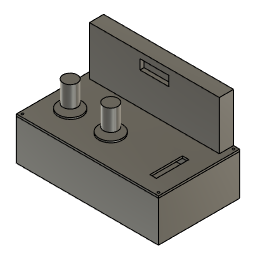
enclosure v8 (Autodesk Fusion 360 design; units mm, degrees)
Autodesk Fusion 360 part; units mm, degrees
note: some values were not read from the file. Set by a fixed rule: which face or edge a step refers to.
sketch "Sketch1" plane through (0, 0, 0) normal (0, 0, 1) x (1, 0, 0) in component "base"
  line L0 (175, 100) -> (-175, 100)
  line L1 (-175, 100) -> (-175, -100)
  line L2 (-175, -100) -> (175, -100)
  line L3 (175, -100) -> (175, 100)
  line L4 (175, 100) -> (-175, -100) construction
  line L5 (-175, 100) -> (175, -100) construction
  dimension "d1" = 350
  dimension "d2" = 200
  constraint horizontal L0
  constraint perpendicular L0 L1
  constraint parallel L0 L2
  constraint parallel L1 L3
  constraint coincident L4 origin
  constraint coincident L5 origin
  measures "d1" distance of L1.end L2.end
  measures "d2" distance of L0.end L1.end
extrude "Extrude1" add sketch "Sketch1" along normal blind 100 makes body 1 in component "base"
sketch "Sketch2" plane through (0, 0, 100) normal (0, 0, 1) x (-1, 0, 0) in component "base"
  line L0 (-175, 100) -> (-175, -100)
  line L1 (-175, -100) -> (175, -100)
  line L2 (175, -100) -> (175, 100)
  line L3 (175, 100) -> (-175, 100)
  line L4 (-160, -85) -> (160, -85)
  line L5 (160, -85) -> (160, 85)
  line L6 (160, 85) -> (-160, 85)
  line L7 (-160, 85) -> (-160, -85)
  line L8 (-160, -85) -> (160, 85) construction
  line L9 (160, -85) -> (-160, 85) construction
  dimension "d5" = 15
  dimension "d6" = 15
  constraint horizontal L4
  constraint perpendicular L4 L5
  constraint parallel L4 L6
  constraint parallel L5 L7
  constraint coincident L8 origin
  constraint coincident L9 origin
  measures "d5" distance of L0 L7
  measures "d6" distance of L3 L6
extrude "Extrude2" cut sketch "Sketch2" against normal up to surface (85 mm away) contours L4 L5 L6 L7 bodies 1 in component "base"
sketch "Sketch3" plane through (0, 0, 100) normal (0, 0, 1) x (-1, 0, 0) in component "base"
  line L0 (-160, 85) -> (160, 85)
  line L1 (160, 85) -> (160, -85)
  line L2 (160, -85) -> (-160, -85)
  line L3 (-160, -85) -> (-160, 85)
  line L4 (-175, 100) -> (-175, -100)
  line L5 (-175, -100) -> (175, -100)
  line L6 (175, -100) -> (175, 100)
  line L7 (175, 100) -> (-175, 100)
  circle A0 centre (-167.5, -92.5) radius 2.5
  dimension "d9" = 7.5
  dimension "d10" = 7.5
  dimension "d11" = 5
  measures "d9" distance of L5 A0.centre
  measures "d10" distance of L4 A0.centre
  measures "d11" diameter of A0
extrude "Extrude3" cut sketch "Sketch3" against normal blind 10 contours A0 bodies 1 in component "base"
mirror "Mirror1" about plane through (0, 0, 0) normal (1, 0, 0) of "Extrude3" in component "base"
mirror "Mirror2" about plane through (0, 0, 0) normal (0, 1, 0) of "Extrude3", "Mirror1" in component "base"
sketch "Sketch1 (2)" plane through (0, 0, 100) normal (0, 0, 1) x (-1, 0, 0) in component "lid"
  circle A0 centre (167.5, 92.5) radius 2.5
  circle A1 centre (-167.5, 92.5) radius 2.5
  circle A2 centre (167.5, -92.5) radius 2.5
  circle A3 centre (-167.5, -92.5) radius 2.5
  line L0 (-160, 85) -> (160, 85)
  line L1 (160, 85) -> (160, -85)
  line L2 (160, -85) -> (-160, -85)
  line L3 (-160, -85) -> (-160, 85)
  line L4 (-175, 100) -> (-175, -100)
  line L5 (-175, -100) -> (175, -100)
  line L6 (175, -100) -> (175, 100)
  line L7 (175, 100) -> (-175, 100)
  line L8 (-175, -100) -> (175, -100)
  line L9 (175, -100) -> (175, 100)
  line L10 (175, 100) -> (-175, 100)
  line L11 (-175, 100) -> (-175, -100)
  line L12 (-175, -100) -> (175, 100) construction
  line L13 (175, -100) -> (-175, 100) construction
  constraint horizontal L8
  constraint perpendicular L8 L9
  constraint parallel L8 L10
  constraint parallel L9 L11
  constraint coincident L12 origin
  constraint coincident L13 origin
  constraint coincident L4.end L5.start
  measures "d109" distance of L4.start
extrude "Extrude1'" add sketch "Sketch1 (2)" along normal blind 5 separate body contours L0 L1 L2 L3 | L4 L5 L6 L7 L8 L9 L10 L11 makes body 2 in component "lid"
sketch "Sketch2 (2)" plane through (0, 0, 105) normal (0, 0, 1) x (-1, 0, 0) in component "lid"
  circle A0 centre (-167.5, -92.5) radius 2.5
  circle A1 centre (167.5, -92.5) radius 2.5
  circle A2 centre (167.5, 92.5) radius 2.5
  circle A3 centre (-167.5, 92.5) radius 2.5
  line L0 (-175, 100) -> (-175, -100)
  line L1 (-175, -100) -> (175, -100)
  line L2 (175, -100) -> (175, 100)
  line L3 (175, 100) -> (-175, 100)
  circle A4 centre (117.5, 25) radius 17.5
  dimension "d20" = 75
  dimension "d21" = 57.5
  dimension "d22" = 35
  measures "d20" distance of L3 A4.centre
  measures "d21" distance of L2 A4.centre
  measures "d22" diameter of A4
extrude "Extrude2'" cut sketch "Sketch2 (2)" against normal blind 5 contours A4 bodies 2 in component "lid"
sketch "Sketch3 (2)" plane through (0, 0, 105) normal (0, 0, 1) x (-1, 0, 0) in component "lid"
  circle A0 centre (117.5, 25) radius 17.5
  circle A1 centre (-167.5, -92.5) radius 2.5
  circle A2 centre (167.5, -92.5) radius 2.5
  circle A3 centre (167.5, 92.5) radius 2.5
  circle A4 centre (-167.5, 92.5) radius 2.5
  line L0 (-175, 100) -> (-175, -100)
  line L1 (-175, -100) -> (175, -100)
  line L2 (175, -100) -> (175, 100)
  line L3 (175, 100) -> (-175, 100)
  circle A5 centre (17.5, 25) radius 17.5
  line L4 (175, 100) -> (-175, 100)
  dimension "d25" = 35
  dimension "d26" = 100
  dimension "d33" = 75
  measures "d25" diameter of A5
  measures "d26" distance of A0.centre A5.centre
  measures "d33" distance of A5.centre L4
extrude "Extrude3'" cut sketch "Sketch3 (2)" against normal blind 5 contours A5 bodies 2 in component "lid"
sketch "Sketch4" plane through (0, 0, 105) normal (0, 0, 1) x (-1, 0, 0) in component "lid"
  circle A0 centre (17.5, 25) radius 17.5
  circle A1 centre (117.5, 25) radius 17.5
  circle A2 centre (-167.5, -92.5) radius 2.5
  circle A3 centre (167.5, -92.5) radius 2.5
  circle A4 centre (167.5, 92.5) radius 2.5
  circle A5 centre (-167.5, 92.5) radius 2.5
  line L0 (-175, 100) -> (-175, -100)
  line L1 (-175, -100) -> (175, -100)
  line L2 (175, -100) -> (175, 100)
  line L3 (175, 100) -> (-175, 100)
  line L4 (-135, 65) -> (-119, 65)
  line L5 (-119, 65) -> (-119, -15)
  line L6 (-119, -15) -> (-135, -15)
  line L7 (-135, -15) -> (-135, 65)
  line L8 (-135, 65) -> (-119, -15) construction
  line L9 (-119, 65) -> (-135, -15) construction
  point P0 (-127, 25)
  dimension "d29" = 40
  dimension "d30" = 80
  dimension "d31" = 16
  dimension "d32" = 35
  constraint horizontal L4
  constraint perpendicular L4 L5
  constraint parallel L4 L6
  constraint parallel L5 L7
  constraint coincident L8 P0
  constraint coincident L9 P0
  measures "d29" distance of L0 L7
  measures "d30" distance of L4.start L6.end
  measures "d31" distance of L5.end L6.end
  measures "d32" distance of L3 L4
extrude "Extrude4" cut sketch "Sketch4" against normal up to surface (5 mm away) contours L4 L5 L6 L7 bodies 2 in component "lid"
sketch "Sketch1 (3)" plane through (0, 0, 105) normal (0, 0, 1) x (-1, 0, 0) in component "display"
  line L0 (-119, -15) -> (-135, -15)
  line L1 (-135, -15) -> (-135, 65)
  line L2 (-135, 65) -> (-119, 65)
  line L3 (-119, 65) -> (-119, -15)
  circle A0 centre (17.5, 25) radius 17.5
  circle A1 centre (117.5, 25) radius 17.5
  circle A2 centre (167.5, 92.5) radius 2.5
  circle A3 centre (-167.5, 92.5) radius 2.5
  circle A4 centre (167.5, -92.5) radius 2.5
  circle A5 centre (-167.5, -92.5) radius 2.5
  line L4 (-175, 100) -> (-175, -100)
  line L5 (-175, -100) -> (175, -100)
  line L6 (175, -100) -> (175, 100)
  line L7 (175, 100) -> (-175, 100)
  line L8 (160, -85) -> (-160, -85)
  line L9 (0, 130) -> (0, -130) construction
  line L10 (-160, -100) -> (160, -100)
  line L11 (160, -100) -> (160, -65)
  line L12 (160, -65) -> (-160, -65)
  line L13 (-160, -65) -> (-160, -100)
  line L14 (-160, -100) -> (160, -65) construction
  line L15 (160, -100) -> (-160, -65) construction
  point P0 (0, -82.5)
  dimension "d36" = 35
  dimension "d37" = 320
  constraint perpendicular L8 L9
  constraint horizontal L10
  constraint perpendicular L10 L11
  constraint parallel L10 L12
  constraint parallel L11 L13
  constraint coincident L14 P0
  constraint coincident L15 P0
  constraint coincident L5 L10.start
  constraint coincident L9 P0
  measures "d36" distance of L10.start L12.end
  measures "d37" distance of L11.end L12.end
extrude "Extrude1''" add sketch "Sketch1 (3)" along normal blind 120 separate body contours L5 L8 L10 L11 L13 | L8 L11 L12 L13 makes body 3 in component "display"
sketch "Sketch1 (4)" plane through (0, 0, 105) normal (0, 0, 1) x (-1, 0, 0) in component "joystick"
  line L0 (-119, -15) -> (-135, -15)
  line L1 (-135, -15) -> (-135, 65)
  line L2 (-135, 65) -> (-119, 65)
  line L3 (-119, 65) -> (-119, -15)
  circle A0 centre (17.5, 25) radius 17.5
  circle A1 centre (117.5, 25) radius 17.5
  circle A2 centre (167.5, 92.5) radius 2.5
  circle A3 centre (-167.5, 92.5) radius 2.5
  circle A4 centre (167.5, -92.5) radius 2.5
  circle A5 centre (-167.5, -92.5) radius 2.5
  line L4 (-175, 100) -> (-175, -100)
  line L5 (-175, -100) -> (175, -100)
  line L6 (175, -100) -> (175, 100)
  line L7 (175, 100) -> (-175, 100)
  circle A6 centre (117.5, 25) radius 29
  dimension "d44" = 58
  constraint concentric A1 A6
  measures "d44" diameter of A6
extrude "Extrude1'''" add sketch "Sketch1 (4)" along normal blind 4 separate body contours A1 | A6 makes body 4 in component "joystick"
sketch "Sketch2 (3)" plane through (0, 0, 109) normal (0, 0, 1) x (-1, 0, 0) in component "joystick"
  circle A0 centre (117.5, 25) radius 29
  circle A1 centre (117.5, 25) radius 3
  dimension "d47" = 6
  constraint concentric A0 A1
  measures "d47" diameter of A1
extrude "Extrude2''" add sketch "Sketch2 (3)" along normal blind 10 contours A1 bodies 4 in component "joystick"
sketch "Sketch3 (3)" plane through (0, 0, 119) normal (0, 0, 1) x (-1, 0, 0) in component "joystick"
  circle A0 centre (117.5, 25) radius 3
  circle A1 centre (117.5, 25) radius 17.5
  dimension "d50" = 35
  constraint concentric A0 A1
  measures "d50" diameter of A1
extrude "Extrude3''" add sketch "Sketch3 (3)" along normal blind 52 contours A0 | A1 bodies 4 in component "joystick"
sketch "Sketch2 (4)" plane through (0, 100, 0) normal (0, 1, 0) x (-1, 0, 0) in component "display"
  line L0 (-160, 105) -> (160, 105)
  line L1 (160, 105) -> (160, 225)
  line L2 (160, 225) -> (-160, 225)
  line L3 (-160, 225) -> (-160, 105)
  line L4 (0, 90) -> (0, 250) construction
  line L5 (145, 220) -> (-145, 220)
  line L6 (-145, 220) -> (-145, 120)
  line L7 (-145, 120) -> (145, 120)
  line L8 (145, 120) -> (145, 220)
  line L9 (145, 220) -> (-145, 120) construction
  line L10 (-145, 220) -> (145, 120) construction
  point P0 (0, 170)
  dimension "d61" = 15
  dimension "d62" = 15
  dimension "d63" = 15
  dimension "d128" = 100
  constraint perpendicular L2 L4
  constraint horizontal L5
  constraint perpendicular L5 L6
  constraint parallel L5 L7
  constraint parallel L6 L8
  constraint coincident L9 P0
  constraint coincident L10 P0
  constraint midpoint L4 P0
  measures "d61" distance of L1 L8
  measures "d62" distance of L3 L6
  measures "d63" distance of L0 L7
  measures "d128" distance of L5.end L6.end
extrude "Extrude2'''" cut sketch "Sketch2 (4)" against normal up to surface (25 mm away) contours L5 L6 L7 L8 bodies 3 in component "display"
sketch "Sketch3 (4)" plane through (0, 75, 0) normal (0, 1, 0) x (-1, 0, 0) in component "display"
  line L0 (145, 220) -> (-145, 220)
  line L1 (-145, 220) -> (-145, 120)
  line L2 (-145, 120) -> (145, 120)
  line L3 (145, 120) -> (145, 220)
  line L4 (0, 80) -> (0, 240) construction
  line L5 (35.5, 210) -> (-35.5, 210)
  line L6 (-35.5, 210) -> (-35.5, 186)
  line L7 (-35.5, 186) -> (35.5, 186)
  line L8 (35.5, 186) -> (35.5, 210)
  line L9 (35.5, 210) -> (-35.5, 186) construction
  line L10 (-35.5, 210) -> (35.5, 186) construction
  point P0 (0, 198)
  dimension "d67" = 10
  dimension "d68" = 24
  dimension "d69" = 71
  constraint vertical L4
  constraint horizontal L5
  constraint perpendicular L5 L6
  constraint parallel L5 L7
  constraint parallel L6 L8
  constraint coincident L9 P0
  constraint coincident L10 P0
  constraint coincident L4 P0
  measures "d67" distance of L0 L5
  measures "d68" distance of L5.end L6.end
  measures "d69" distance of L5.start L5.end
extrude "Extrude3'''" cut sketch "Sketch3 (4)" against normal up to surface (10 mm away) contours L5 L6 L7 L8 bodies 3 in component "display"
sketch "Sketch5" plane through (0, 100, 0) normal (0, 1, 0) x (-1, 0, 0)
  line L0 (145, 120) -> (-145, 120)
  line L1 (-145, 120) -> (-145, 220)
  line L2 (-145, 220) -> (145, 220)
  line L3 (145, 220) -> (145, 120)
  line L4 (-160, 105) -> (160, 105)
  line L5 (160, 105) -> (160, 225)
  line L6 (160, 225) -> (-160, 225)
  line L7 (-160, 225) -> (-160, 105)
  line L8 (-35.5, 186) -> (-35.5, 210)
  line L9 (-47.4876, 205) -> (45, 205) construction
  line L10 (-35.5, 210) -> (14.5, 210)
  line L11 (14.5, 210) -> (14.5, 227)
  line L12 (14.5, 227) -> (-35.5, 227)
  line L13 (-35.5, 227) -> (-35.5, 210)
  dimension "d76" = 50
  dimension "d77" = 17
  constraint perpendicular L8 L9
  constraint horizontal L10
  constraint vertical L11
  constraint horizontal L12
  constraint vertical L13
  constraint coincident L8.end L10.start
  measures "d76" distance of L11.end L12.end
  measures "d77" distance of L10.end L11.end
sketch "Sketch6" plane through (0, 75, 0) normal (0, 1, 0) x (-1, 0, 0)
  line L0 (-35.5, 186) -> (-35.5, 210)
  line L1 (-145, 220) -> (-145, 120)
  line L2 (-145, 120) -> (145, 120)
  line L3 (145, 120) -> (145, 220)
  line L4 (145, 220) -> (-145, 220)
  line L5 (-35.5, 210) -> (35.5, 210)
  line L6 (35.5, 210) -> (35.5, 186)
  line L7 (35.5, 186) -> (-35.5, 186)
  circle A0 centre (37.5, 213) radius 1.5
  dimension "d80" = 2
  dimension "d81" = 3
  dimension "d82" = 3
  measures "d80" distance of L6 A0.centre
  measures "d81" distance of L5 A0.centre
  measures "d82" diameter of A0
extrude "Extrude5" cut sketch "Sketch6" against normal up to surface (5 mm away) contours A0 bodies 3 in component "display"
ref_plane "WorkPlane1" through (0, 70, 198) normal (0, 0, 1) x (-1, 0, 0)
mirror "Mirror1'" about plane through (0, 70, 198) normal (0, 0, 1) of "Extrude5" in component "display"
mirror "Mirror2'" about plane through (0, 0, 0) normal (1, 0, 0) of "Extrude5", "Mirror1'" in component "display"
sketch "Sketch4 (2)" plane through (0, 0, 100) normal (0, 0, 1) x (-1, 0, 0) in component "base"
  circle A0 centre (167.5, 92.5) radius 2.5
  circle A1 centre (-167.5, 92.5) radius 2.5
  circle A2 centre (167.5, -92.5) radius 2.5
  circle A3 centre (-167.5, -92.5) radius 2.5
  line L0 (-160, 85) -> (160, 85)
  line L1 (160, 85) -> (160, -85)
  line L2 (160, -85) -> (-160, -85)
  line L3 (-160, -85) -> (-160, 85)
  line L4 (-175, 100) -> (-175, -100)
  line L5 (-175, -100) -> (175, -100)
  line L6 (175, -100) -> (175, 100)
  line L7 (175, 100) -> (-175, 100)
  line L8 (188.1684, -92.5) -> (-190, -92.5) construction
  circle A4 centre (105, -92.5) radius 2.5
  dimension "d91" = 5
  dimension "d92" = 70
  constraint perpendicular L4 L8
  constraint coincident L8 A4.centre
  measures "d91" diameter of A4
  measures "d92" distance of L6 A4.centre
extrude "Extrude4'" cut sketch "Sketch4 (2)" against normal blind 10 contours A4 bodies 1 in component "base"
mirror "Mirror3" about plane through (0, 0, 0) normal (1, 0, 0) of "Extrude4'" in component "base"
sketch "Sketch5 (2)" plane through (0, 0, 105) normal (0, 0, 1) x (-1, 0, 0) in component "lid"
  line L0 (-119, -15) -> (-135, -15)
  line L1 (-135, -15) -> (-135, 65)
  line L2 (-135, 65) -> (-119, 65)
  line L3 (-119, 65) -> (-119, -15)
  circle A0 centre (17.5, 25) radius 17.5
  circle A1 centre (117.5, 25) radius 17.5
  circle A2 centre (167.5, 92.5) radius 2.5
  circle A3 centre (-167.5, 92.5) radius 2.5
  circle A4 centre (167.5, -92.5) radius 2.5
  circle A5 centre (-167.5, -92.5) radius 2.5
  line L4 (-175, 100) -> (-175, -100)
  line L5 (-175, -100) -> (175, -100)
  line L6 (175, -100) -> (175, 100)
  line L7 (175, 100) -> (-175, 100)
  circle A6 centre (-105, -92.5) radius 2.5
  circle A7 centre (-105, -92.5) radius 2.5
  dimension "d97" = 5
  constraint concentric A6 A7
  measures "d97" diameter of A6
extrude "Extrude5'" cut sketch "Sketch5 (2)" against normal up to surface (5 mm away) contours A6 A7 bodies 2 in component "lid"
sketch "Sketch4 (3)" plane through (0, 0, 120) normal (0, 0, 1) x (-1, 0, 0) in component "display"
  line L0 (145, -75) -> (-145, -75)
  line L1 (-145, -75) -> (-145, -100)
  line L2 (-145, -100) -> (145, -100)
  line L3 (145, -100) -> (145, -75)
  circle A0 centre (-105, -92.5) radius 2.5
  circle A1 centre (105, -92.5) radius 2.5
  point P0 (-175, -100)
  point P1 (175, -100)
  dimension "d100" = 5
  dimension "d101" = 5
  dimension "d102" = 70
  dimension "d103" = 70
  dimension "d120" = 7.5
  dimension "d121" = 7.5
  measures "d100" diameter of A1
  measures "d101" diameter of A0
  measures "d102" horizontal distance of A0.centre P0
  measures "d103" horizontal distance of A1.centre P1
  measures "d120" distance of L2 A1.centre
  measures "d121" distance of L2 A0.centre
extrude "Extrude6" cut sketch "Sketch4 (3)" against normal up to surface (15 mm away) contours A0 | A1 bodies 3 in component "display"
mirror "Mirror1''" about plane through (0, 0, 0) normal (1, 0, 0) of "Extrude5'" in component "lid"
sketch "Sketch5 (3)" plane through (0, 75, 0) normal (0, 1, 0) x (-1, 0, 0) in component "display"
  circle A0 centre (-37.5, 213) radius 1.5
  circle A1 centre (37.5, 183) radius 1.5
  circle A2 centre (37.5, 213) radius 1.5
  line L0 (-35.5, 186) -> (-35.5, 210)
  line L1 (-145, 220) -> (-145, 120)
  line L2 (-145, 120) -> (145, 120)
  line L3 (145, 120) -> (145, 220)
  line L4 (145, 220) -> (-145, 220)
  line L5 (-35.5, 210) -> (35.5, 210)
  line L6 (35.5, 210) -> (35.5, 186)
  line L7 (35.5, 186) -> (-35.5, 186)
  line L8 (-145, 120) -> (-135, 120)
  line L9 (-135, 120) -> (-135, 130)
  line L10 (-135, 130) -> (-145, 130)
  line L11 (-145, 130) -> (-145, 120)
  circle A3 centre (-37.5, 183) radius 1.5
  dimension "d108" = 10
  dimension "d109" = 10
  constraint horizontal L8
  constraint vertical L9
  constraint horizontal L10
  constraint vertical L11
  constraint coincident L1.end L2.start
  measures "d108" distance of L9.end L10.end
  measures "d109" distance of L8.end L9.end
extrude "Extrude7" add sketch "Sketch5 (3)" along normal up to surface (20 mm away) contours L1 L2 L8 L9 L10 L11 bodies 3 in component "display"
sketch "Sketch6 (2)" plane through (0, 95, 0) normal (0, 1, 0) x (-1, 0, 0) in component "display"
  line L0 (-135, 130) -> (-145, 130)
  line L1 (-145, 130) -> (-145, 120)
  line L2 (-145, 120) -> (-135, 120)
  line L3 (-135, 120) -> (-135, 130)
  circle A0 centre (-140, 125) radius 2.5
  dimension "d117" = 5
  measures "d117" diameter of A0
extrude "Extrude8" cut sketch "Sketch6 (2)" against normal blind 10 contours A0 bodies 3 in component "display"
mirror "Mirror3'" about plane through (0, 0, 0) normal (1, 0, 0) of "Extrude7", "Extrude8" in component "display"
ref_plane "WorkPlane1" through (0, 87.5, 167.5) normal (0, 0, 1) x (-1, 0, 0) in component "display"
mirror "Mirror4" about plane through (0, 87.5, 167.5) normal (0, 0, 1) of "Extrude7", "Extrude8", "Mirror3'" in component "display"
sketch "Sketch1 (5)" plane through (0, 100, 0) normal (0, 1, 0) x (-1, 0, 0) in component "display back piece"
  line L0 (-160, 105) -> (160, 105)
  line L1 (160, 105) -> (160, 225)
  line L2 (160, 225) -> (-160, 225)
  line L3 (-160, 225) -> (-160, 105)
  line L4 (145, 220) -> (145, 120)
  line L5 (145, 120) -> (-145, 120)
  line L6 (-145, 120) -> (-145, 220)
  line L7 (-145, 220) -> (145, 220)
  line L8 (-145, 220) -> (145, 220)
  line L9 (145, 220) -> (145, 120)
  line L10 (145, 120) -> (-145, 120)
  line L11 (-145, 120) -> (-145, 220)
  constraint horizontal L8
  constraint vertical L9
  constraint horizontal L10
  constraint vertical L11
  constraint coincident L4.end L5.start
  constraint coincident L6.end L7.start
extrude "Extrude1''''" add sketch "Sketch1 (5)" against normal up to surface (5 mm away) separate body contours L4 L5 L6 L7 L8 L9 L10 L11 makes body 5 in component "display back piece"
sketch "Sketch2 (5)" plane through (0, 100, 0) normal (0, 1, 0) x (-1, 0, 0) in component "display back piece"
  line L0 (-145, 120) -> (145, 120)
  line L1 (145, 120) -> (145, 220)
  line L2 (145, 220) -> (-145, 220)
  line L3 (-145, 220) -> (-145, 120)
  circle A0 centre (-140, 210) radius 2.5
extrude "Extrude2''''" cut sketch "Sketch2 (5)" against normal blind 5 contours A0 bodies 5 in component "display back piece"
mirror "Mirror1'''" about plane through (0, 0, 0) normal (1, 0, 0) of "Extrude2''''" in component "display back piece"
mirror "Mirror2''" about plane through (0, 87.5, 167.5) normal (0, 0, 1) of 2 faces at (139.3229, 96.6667, 212.4066) (-139.3229, 96.6667, 212.4066) on bodies 5 in component "display back piece"
sketch "Sketch8" plane through (0, 75, 0) normal (0, 1, 0) x (-1, 0, 0)
  circle A0 centre (-37.5, 183) radius 1.5
  circle A1 centre (-37.5, 213) radius 1.5
  circle A2 centre (37.5, 183) radius 1.5
  circle A3 centre (37.5, 213) radius 1.5
  line L0 (35.5, 186) -> (-35.5, 186)
  line L1 (-35.5, 186) -> (-35.5, 210)
  line L2 (-35.5, 210) -> (35.5, 210)
  line L3 (35.5, 210) -> (35.5, 186)
  line L4 (145, 205) -> (135, 205)
  line L5 (135, 205) -> (135, 215)
  line L6 (135, 215) -> (145, 215)
  line L7 (145, 215) -> (145, 220)
  line L8 (145, 220) -> (-145, 220)
  line L9 (-145, 220) -> (-145, 215)
  line L10 (-145, 215) -> (-135, 215)
  line L11 (-135, 215) -> (-135, 205)
  line L12 (-135, 205) -> (-145, 205)
  line L13 (-145, 205) -> (-145, 130)
  line L14 (-145, 130) -> (-135, 130)
  line L15 (-135, 130) -> (-135, 120)
  line L16 (-135, 120) -> (135, 120)
  line L17 (135, 120) -> (135, 130)
  line L18 (135, 130) -> (145, 130)
  line L19 (145, 130) -> (145, 205)
  line L20 (-35.5, 210) -> (35.5, 210)
  line L21 (35.5, 210) -> (35.5, 220)
  line L22 (35.5, 220) -> (-35.5, 220)
  line L23 (-35.5, 220) -> (-35.5, 210)
  constraint horizontal L20
  constraint vertical L21
  constraint horizontal L22
  constraint vertical L23
  constraint coincident L8 L21.end
  constraint coincident L1.end L2.start
extrude "Extrude9" cut sketch "Sketch8" against normal up to surface (8 mm away) contours L2 L8 L20 L21 L22 L23 bodies 3 in component "display"
sketch "Sketch7" plane through (0, 0, 120) normal (0, 0, 1) x (-1, 0, 0) in component "display"
  circle A0 centre (105, -92.5) radius 2.5
  circle A1 centre (-105, -92.5) radius 2.5
  line L0 (145, -95) -> (135, -95)
  line L1 (135, -95) -> (135, -75)
  line L2 (135, -75) -> (-135, -75)
  line L3 (-135, -75) -> (-135, -95)
  line L4 (-135, -95) -> (-145, -95)
  line L5 (-145, -95) -> (-145, -100)
  line L6 (-145, -100) -> (145, -100)
  line L7 (145, -100) -> (145, -95)
  line L8 (0, -75) -> (0, -120) construction
  line L9 (10, -75) -> (-10, -75)
  line L10 (-10, -75) -> (-10, -85)
  line L11 (-10, -85) -> (10, -85)
  line L12 (10, -85) -> (10, -75)
  line L13 (10, -75) -> (-10, -85) construction
  line L14 (-10, -75) -> (10, -85) construction
  point P0 (0, -80)
  dimension "d138" = 10
  dimension "d139" = 20
  constraint midpoint L2 L8.start
  constraint perpendicular L6 L8
  constraint horizontal L9
  constraint perpendicular L9 L10
  constraint parallel L9 L11
  constraint parallel L10 L12
  constraint coincident L13 P0
  constraint coincident L14 P0
  constraint coincident L2 L9.start
  constraint coincident L8 P0
  measures "d138" distance of L9.start L11.end
  measures "d139" distance of L10.end L11.end
extrude "Extrude10" cut sketch "Sketch7" against normal up to surface (15 mm away) contours L2 L9 L10 L11 L12 bodies 3 in component "display"
sketch "Sketch6 (3)" plane through (0, 0, 105) normal (0, 0, 1) x (-1, 0, 0) in component "lid"
  circle A0 centre (105, -92.5) radius 2.5
  circle A1 centre (-105, -92.5) radius 2.5
  line L0 (-119, -15) -> (-135, -15)
  line L1 (-135, -15) -> (-135, 65)
  line L2 (-135, 65) -> (-119, 65)
  line L3 (-119, 65) -> (-119, -15)
  circle A2 centre (17.5, 25) radius 17.5
  circle A3 centre (117.5, 25) radius 17.5
  circle A4 centre (167.5, 92.5) radius 2.5
  circle A5 centre (-167.5, 92.5) radius 2.5
  circle A6 centre (167.5, -92.5) radius 2.5
  circle A7 centre (-167.5, -92.5) radius 2.5
  line L4 (-175, 100) -> (-175, -100)
  line L5 (-175, -100) -> (175, -100)
  line L6 (175, -100) -> (175, 100)
  line L7 (175, 100) -> (-175, 100)
  line L8 (0, -140) -> (0, -30) construction
  line L9 (-10, -85) -> (10, -85)
  line L10 (10, -85) -> (10, -75)
  line L11 (10, -75) -> (-10, -75)
  line L12 (-10, -75) -> (-10, -85)
  line L13 (-10, -85) -> (10, -75) construction
  line L14 (10, -85) -> (-10, -75) construction
  line L15 (-175, -100) -> (175, -100)
  point P0 (0, -80)
  dimension "d142" = 10
  dimension "d143" = 20
  dimension "d144" = 15
  constraint vertical L8
  constraint horizontal L9
  constraint perpendicular L9 L10
  constraint parallel L9 L11
  constraint parallel L10 L12
  constraint coincident L13 P0
  constraint coincident L14 P0
  constraint coincident L8 P0
  measures "d142" distance of L9.start L11.end
  measures "d143" distance of L10.end L11.end
  measures "d144" distance of L9 L15
extrude "Extrude6'" cut sketch "Sketch6 (3)" against normal up to surface (5 mm away) contours L9 L10 L11 L12 bodies 2 in component "lid"
component "base" placed x (1, 0, 0) y (0, 1, 0) z (0, 0, 1) at (0, 0, 0)
component "lid" placed x (1, 0, 0) y (0, 1, 0) z (0, 0, 1) at (0, 0, 0)
component "display" placed x (1, 0, 0) y (0, 1, 0) z (0, 0, 1) at (0, 0, 0)
component "joystick" placed x (1, 0, 0) y (0, 1, 0) z (0, 0, 1) at (0, 0, 0)
component "joystick" placed x (1, 0, 0) y (0, 1, 0) z (0, 0, 1) at (100, 0, 0)
component "display back piece" placed x (1, 0, 0) y (0, 1, 0) z (0, 0, 1) at (0, 0, 0)
